Autodesk Fusion 360 part; units mm, degrees
note: some values were not read from the file. Set by a fixed rule: which sketch regions a step uses.
(part 3 of 8)
  line L1327 (107.274, 60.7841) -> (107.274, 61.6082)
  line L1328 (90.83, 67.0833) -> (104.831, 67.0833)
  line L1329 (38.442, 33.0844) -> (37.642, 33.0844)
  line L1330 (124.167, 80.0836) -> (123.367, 80.0836)
  line L1331 (100.355, 105.5592) -> (99.556, 105.5592)
  line L1332 (80.506, 108.6602) -> (81.305, 108.6602)
  line L1333 (138.167, 81.084) -> (124.167, 81.084)
  line L1334 (124.167, 76.9844) -> (123.367, 76.9844)
  line L1335 (38.442, 38.8844) -> (37.642, 38.8844)
  line L1336 (95.306, 108.6602) -> (96.105, 108.6602)
  line L1337 (81.305, 99.7592) -> (80.506, 99.7592)
  line L1338 (37.642, 38.8844) -> (37.642, 41.9836)
  line L1339 (115.155, 108.6602) -> (114.356, 108.6602)
  line L1340 (80.506, 105.5592) -> (81.305, 105.5592)
  line L1341 (100.355, 109.6602) -> (114.356, 109.6602)
  line L1342 (142.417, 105.5592) -> (143.217, 105.5592)
  line L1343 (123.367, 68.0838) -> (123.367, 71.1844)
  line L1344 (37.642, 41.9836) -> (37.642, 38.8844)
  line L1345 (95.306, 108.6602) -> (95.306, 109.6602)
  line L1346 (81.305, 96.6592) -> (81.305, 95.6582)
  line L1347 (38.442, 29.9838) -> (37.642, 29.9838)
  line L1348 (100.355, 108.6602) -> (100.355, 109.6602)
  line L1349 (96.105, 108.6602) -> (96.105, 105.5592)
  line L1350 (90.031, 71.1844) -> (90.83, 71.1844)
  arc A24 (90.274, 120.9832) -> (88.274, 118.9832) centre (90.274, 118.9832) ccw
  line L1351 (110.974, 53.3084) -> (110.974, 52.509)
  line L1352 (90.031, 68.0838) -> (90.031, 71.1844)
  line L1353 (95.306, 109.6602) -> (95.306, 108.6602)
  line L1354 (96.105, 105.5592) -> (95.306, 105.5592)
  line L1355 (80.506, 99.7592) -> (80.506, 96.6592)
  line L1356 (100.355, 109.6602) -> (100.355, 108.6602)
  circle A25 centre (99.974, 117.5832) radius 1.7
  arc A26 (86.274, 114.1832) -> (88.274, 116.1832) centre (86.274, 116.1832) ccw
  line L1357 (81.305, 96.6592) -> (80.506, 96.6592)
  line L1358 (81.305, 95.6582) -> (81.305, 96.6592)
  line L1359 (115.155, 108.6602) -> (115.155, 105.5592)
  line L1360 (138.968, 96.6592) -> (138.968, 99.7592)
  line L1361 (89.306, 67.3134) -> (87.581, 67.3134)
  line L1362 (90.83, 71.1844) -> (90.83, 71.7838)
  line L1363 (100.355, 108.6602) -> (99.556, 108.6602)
  line L1364 (102.673, 52.509) -> (102.673, 54.0334)
  line L1365 (114.356, 109.6602) -> (100.355, 109.6602)
  line L1366 (90.83, 67.0833) -> (90.83, 68.0838)
  line L1367 (104.474, 61.6082) -> (104.474, 60.7841)
  line L1368 (43.718, 22.9336) -> (42.917, 22.9336)
  line L1369 (97.974, 52.509) -> (98.973, 52.509)
  line L1370 (90.031, 71.1844) -> (90.031, 68.0838)
  line L1371 (43.718, 22.9336) -> (43.718, 19.8345)
  line L1372 (111.674, 118.9832) -> (111.674, 116.1832)
  line L1373 (90.83, 71.7838) -> (89.306, 71.7838)
  line L1374 (81.305, 108.6602) -> (81.305, 109.6602)
  line L1375 (42.917, 22.9336) -> (42.917, 23.934)
  line L1376 (98.204, 59.0591) -> (98.204, 60.7841)
  line L1377 (138.968, 108.6602) -> (138.968, 105.5592)
  line L1378 (81.305, 99.7592) -> (81.305, 105.5592)
  line L1379 (98.204, 59.0591) -> (97.224, 59.0591)
  line L1380 (28.117, 22.9336) -> (28.917, 22.9336)
  line L1381 (90.031, 68.0838) -> (90.83, 68.0838)
  line L1382 (143.217, 108.6602) -> (143.217, 109.6602)
  line L1383 (81.305, 108.6602) -> (80.506, 108.6602)
  line L1384 (80.506, 99.7592) -> (81.305, 99.7592)
  line L1385 (109.674, 120.9832) -> (90.274, 120.9832)
  line L1386 (81.305, 109.6602) -> (81.305, 108.6602)
  line L1387 (80.506, 108.6602) -> (80.506, 105.5592)
  line L1388 (87.581, 66.3337) -> (87.581, 67.3134)
  line L1389 (142.417, 96.6592) -> (143.217, 96.6592)
  line L1390 (114.356, 105.5592) -> (115.155, 105.5592)
  line L1391 (95.306, 105.5592) -> (96.105, 105.5592)
  line L1392 (138.167, 105.5592) -> (138.968, 105.5592)
  line L1393 (114.356, 108.6602) -> (114.356, 109.6602)
  line L1394 (104.474, 60.7841) -> (98.204, 60.7841)
  line L1395 (138.968, 108.6602) -> (138.167, 108.6602)
  line L1396 (95.306, 95.6582) -> (81.305, 95.6582)
  line L1397 (96.105, 108.6602) -> (95.306, 108.6602)
  line L1398 (28.917, 23.934) -> (28.917, 22.9336)
  arc A27 (181.673, -20.7426) -> (183.673, -18.7426) centre (181.673, -18.7426) ccw
  line L1399 (80.506, 96.6592) -> (81.305, 96.6592)
  arc A28 (224.567, -18.7426) -> (226.567, -20.7426) centre (226.567, -18.7426) ccw
  line L1400 (89.306, 67.3134) -> (89.306, 71.7838)
  circle A29 centre (171.973, -17.3426) radius 1.7
  line L1401 (90.83, 68.0838) -> (90.83, 67.0833)
  line L1402 (138.167, 95.6582) -> (138.167, 96.6592)
  line L1403 (102.673, 52.509) -> (102.073, 52.509)
  line L1404 (143.217, 68.0838) -> (143.217, 67.0833)
  line L1405 (138.167, 96.6592) -> (138.968, 96.6592)
  line L1406 (99.556, 105.5592) -> (99.556, 108.6602)
  line L1407 (84.28, 66.3337) -> (87.581, 66.3337)
  line L1408 (89.306, 71.7838) -> (89.306, 67.3134)
  line L1409 (42.917, 19.8345) -> (43.718, 19.8345)
  line L1410 (43.718, 19.8345) -> (42.917, 19.8345)
  line L1411 (143.217, 108.6602) -> (142.417, 108.6602)
  line L1412 (100.374, 120.9832) -> (99.574, 120.9832)
  line L1413 (98.973, 52.509) -> (98.973, 53.3084)
  line L1414 (88.274, 118.9832) -> (88.274, 116.1832)
  line L1415 (28.917, 22.9336) -> (28.117, 22.9336)
  arc A30 (245.967, -20.7426) -> (247.967, -18.7426) centre (245.967, -18.7426) ccw
  line L1416 (87.581, 66.3337) -> (84.28, 66.3337)
  line L1417 (96.105, 105.5592) -> (96.105, 108.6602)
  line L1418 (42.917, 23.934) -> (42.917, 22.9336)
  line L1419 (143.217, 109.6602) -> (143.217, 108.6602)
  line L1420 (142.417, 71.1844) -> (142.417, 68.0838)
  arc A31 (160.273, -15.9426) -> (158.273, -13.9426) centre (158.273, -15.9426) ccw
  line L1421 (81.305, 95.6582) -> (95.306, 95.6582)
  line L1422 (87.581, 67.3134) -> (87.581, 66.3337)
  line L1423 (81.731, 76.3836) -> (82.555, 76.3836)
  line L1424 (47.681, 61.0336) -> (47.681, 62.034)
  line L1425 (82.555, 67.3134) -> (84.28, 67.3134)
  line L1426 (24.668, 22.9336) -> (24.668, 19.8345)
  line L1427 (51.931, 49.0338) -> (52.73, 49.0338)
  line L1428 (-119.0079, 28.9833) -> (-133.0076, 28.9833)
  line L1429 (24.668, 19.8345) -> (23.867, 19.8345)
  line L1430 (48.48, 52.1344) -> (47.681, 52.1344)
  line L1431 (23.867, 22.9336) -> (23.867, 23.934)
  line L1432 (82.555, 79.6137) -> (82.555, 76.3836)
  line L1433 (8.724, 0.1836) -> (-30.902, 0.1836)
  arc A32 (-163.6637, -15.9426) -> (-165.6637, -13.9426) centre (-165.6637, -15.9426) ccw
  line L1434 (24.668, 22.9336) -> (23.867, 22.9336)
  arc A33 (-147.2637, -20.7426) -> (-145.2637, -18.7426) centre (-147.2637, -18.7426) ccw
  line L1435 (-18.994, 81.084) -> (-32.995, 81.084)
  line L1436 (23.867, 19.8345) -> (24.668, 19.8345)
  line L1437 (47.681, 52.1344) -> (47.681, 57.9344)
  line L1438 (77.055, 68.0838) -> (77.055, 71.1844)
  line L1439 (47.681, 61.0336) -> (48.48, 61.0336)
  line L1440 (-140.1512, -9.1167) -> (-126.1517, -9.1167)
  line L1441 (-145.2637, -18.7426) -> (-145.2637, -15.9426)
  line L1442 (76.256, 71.1844) -> (76.256, 76.9844)
  arc A34 (-106.601, -18.7426) -> (-104.601, -20.7426) centre (-104.601, -18.7426) ccw
  line L1443 (24.668, 19.8345) -> (24.668, 22.9336)
  line L1444 (-133.0076, 28.9833) -> (-119.0079, 28.9833)
  line L1445 (81.731, 73.5836) -> (82.555, 73.5836)
  line L1446 (51.931, 57.9344) -> (51.931, 61.0336)
  line L1447 (77.055, 80.0836) -> (76.256, 80.0836)
  line L1448 (-23.47, 62.034) -> (-9.469, 62.034)
  line L1449 (23.867, 23.934) -> (23.867, 22.9336)
  line L1450 (81.731, 76.3836) -> (81.731, 73.5836)
  arc A35 (-106.601, -15.9426) -> (-108.601, -13.9426) centre (-108.601, -15.9426) ccw
  line L1451 (-142.5325, 23.934) -> (-128.5329, 23.934)
  circle A36 centre (-156.9637, -17.3426) radius 1.7
  line L1452 (-18.994, 67.0833) -> (-32.995, 67.0833)
  line L1453 (-128.5329, 9.9333) -> (-142.5325, 9.9333)
  circle A37 centre (-156.9637, -17.3426) radius 1.7
  line L1454 (19.392, 42.984) -> (33.392, 42.984)
  line L1455 (-165.6637, -13.9426) -> (-171.0689, -13.9426)
  arc A38 (-163.6637, -18.7426) -> (-161.6637, -20.7426) centre (-161.6637, -18.7426) ccw
  line L1456 (-123.769, 62.034) -> (-137.77, 62.034)
  line L1457 (28.631, 57.9344) -> (29.43, 57.9344)
  line L1458 (23.867, 22.9336) -> (24.668, 22.9336)
  line L1459 (-4.708, 28.9833) -> (-18.708, 28.9833)
  line L1460 (-126.1517, -9.1167) -> (-140.1512, -9.1167)
  line L1461 (-32.995, 67.0833) -> (-18.994, 67.0833)
  line L1462 (261.656, -7.9426) -> (261.656, 108.1832)
  circle A39 centre (-94.901, -17.3426) radius 1.7
  line L1463 (-126.1517, 4.8841) -> (-140.1512, 4.8841)
  line L1464 (28.631, 49.0338) -> (28.631, 48.0333)
  line L1465 (-133.0076, 42.984) -> (-119.0079, 42.984)
  line L1466 (-119.0079, 42.984) -> (-133.0076, 42.984)
  line L1467 (19.392, 28.9833) -> (33.392, 28.9833)
  line L1468 (33.392, 28.9833) -> (19.392, 28.9833)
  line L1469 (33.392, 42.984) -> (19.392, 42.984)
  line L1470 (-18.708, 42.984) -> (-4.708, 42.984)
  line L1471 (-114.244, 67.0833) -> (-128.2451, 67.0833)
  arc A40 (-143.2637, -13.9426) -> (-145.2637, -15.9426) centre (-143.2637, -15.9426) ccw
  line L1472 (29.43, 49.0338) -> (28.631, 49.0338)
  line L1473 (5.398, -13.9426) -> (-81.201, -13.9426)
  line L1474 (33.68, 52.1344) -> (33.68, 57.9344)
  line L1475 (-108.601, -13.9426) -> (-143.2637, -13.9426)
  line L1476 (-150.5637, -13.9426) -> (-101.301, -13.9426)
  circle A41 centre (-94.901, -17.3426) radius 1.7
  line L1477 (-106.601, -18.7426) -> (-106.601, -15.9426)
  line L1478 (195.605, -9.1167) -> (209.607, -9.1167)
  line L1479 (219.132, 41.9836) -> (219.132, 42.984)
  line L1480 (157.217, 22.9336) -> (157.217, 23.934)
  line L1481 (0.342, 29.9838) -> (0.342, 28.9833)
  line L1482 (32.881, 52.1344) -> (33.68, 52.1344)
  line L1483 (28.631, 61.0336) -> (28.631, 62.034)
  line L1484 (158.018, 22.9336) -> (157.217, 22.9336)
  line L1485 (32.881, 57.9344) -> (32.881, 61.0336)
  line L1486 (28.631, 52.1344) -> (29.43, 52.1344)
  line L1487 (-95.301, -20.7426) -> (-94.501, -20.7426)
  line L1488 (-163.6637, -18.7426) -> (-163.6637, -15.9426)
  line L1489 (32.881, 52.1344) -> (32.881, 49.0338)
  line L1490 (157.217, 14.0343) -> (157.217, 19.8345)
  line L1491 (29.43, 49.0338) -> (29.43, 52.1344)
  line L1492 (32.881, 57.9344) -> (33.68, 57.9344)
  line L1493 (185.673, 114.1832) -> (222.567, 114.1832)
  line L1494 (157.217, 22.9336) -> (158.018, 22.9336)
  line L1495 (157.217, 14.0343) -> (158.018, 14.0343)
  line L1496 (29.43, 52.1344) -> (28.631, 52.1344)
  line L1497 (-114.244, 81.084) -> (-128.2451, 81.084)
  line L1498 (158.018, 19.8345) -> (158.018, 22.9336)
  line L1499 (33.68, 48.0333) -> (33.68, 49.0338)
  line L1500 (0.342, 38.8844) -> (0.342, 33.0844)
  line L1501 (158.018, 14.0343) -> (158.018, 10.9337)
  line L1502 (32.881, 49.0338) -> (33.68, 49.0338)
  line L1503 (157.217, 10.9337) -> (158.018, 10.9337)
  line L1504 (-9.469, 95.6582) -> (-23.47, 95.6582)
  line L1505 (219.132, 33.0844) -> (219.132, 38.8844)
  line L1506 (29.43, 57.9344) -> (29.43, 61.0336)
  line L1507 (-99.6701, 62.034) -> (-99.6701, 61.0336)
  line L1508 (238.182, -9.1167) -> (224.18, -9.1167)
  line L1509 (32.881, 49.0338) -> (32.881, 52.1344)
  line L1510 (-100.4691, 61.0336) -> (-100.4691, 57.9344)
  line L1511 (158.018, 19.8345) -> (157.217, 19.8345)
  line L1512 (-9.469, 62.034) -> (-23.47, 62.034)
  line L1513 (186.08, 33.0844) -> (185.279, 33.0844)
  line L1514 (-0.458, 29.9838) -> (0.342, 29.9838)
  line L1515 (158.018, 10.9337) -> (157.217, 10.9337)
  line L1516 (-103.92, 52.1344) -> (-103.92, 49.0338)
  line L1517 (158.018, 10.9337) -> (158.018, 14.0343)
  line L1518 (-103.92, 49.0338) -> (-103.92, 52.1344)
  line L1519 (0.342, 42.984) -> (0.342, 41.9836)
  line L1520 (219.132, 38.8844) -> (219.132, 33.0844)
  line L1521 (158.018, 22.9336) -> (158.018, 19.8345)
  line L1522 (157.217, 23.934) -> (157.217, 22.9336)
  line L1523 (28.631, 49.0338) -> (29.43, 49.0338)
  line L1524 (161.467, 61.0336) -> (161.467, 57.9344)
  line L1525 (186.08, 38.8844) -> (185.279, 38.8844)
  line L1526 (-100.4691, 57.9344) -> (-100.4691, 61.0336)
  line L1527 (-103.92, 57.9344) -> (-103.92, 61.0336)
  line L1528 (194.804, 3.8837) -> (194.804, 0.7845)
  line L1529 (32.881, 61.0336) -> (32.881, 57.9344)
  line L1530 (29.43, 61.0336) -> (29.43, 57.9344)
  line L1531 (-0.458, 38.8844) -> (-0.458, 41.9836)
  line L1532 (-28.233, 9.9333) -> (-14.233, 9.9333)
  line L1533 (0.342, 29.9838) -> (-0.458, 29.9838)
  line L1534 (0.342, 33.0844) -> (-0.458, 33.0844)
  line L1535 (192.356, 4.3343) -> (192.356, 3.4138)
  line L1536 (161.467, 49.0338) -> (161.467, 52.1344)
  line L1537 (-104.719, 48.0333) -> (-104.719, 49.0338)
  line L1538 (-100.4691, 52.1344) -> (-100.4691, 49.0338)
  line L1539 (33.68, 49.0338) -> (33.68, 48.0333)
  line L1540 (157.217, 49.0338) -> (157.217, 48.0333)
  line L1541 (158.018, 49.0338) -> (158.018, 52.1344)
  line L1542 (157.217, 19.8345) -> (158.018, 19.8345)
  line L1543 (-103.92, 61.0336) -> (-103.92, 57.9344)
  line L1544 (157.217, 10.9337) -> (157.217, 9.9333)
  line L1545 (185.279, 38.8844) -> (185.279, 41.9836)
  line L1546 (157.217, 9.9333) -> (157.217, 10.9337)
  line L1547 (-0.458, 41.9836) -> (0.342, 41.9836)
  line L1548 (33.68, 57.9344) -> (33.68, 52.1344)
  line L1549 (-0.458, 33.0844) -> (-0.458, 29.9838)
  line L1550 (33.68, 61.0336) -> (32.881, 61.0336)
  line L1551 (157.217, 48.0333) -> (157.217, 49.0338)
  line L1552 (-0.458, 41.9836) -> (-0.458, 38.8844)
  line L1553 (28.631, 61.0336) -> (29.43, 61.0336)
  line L1554 (-100.4691, 52.1344) -> (-99.6701, 52.1344)
  line L1555 (192.356, 3.4138) -> (192.356, 4.3343)
  line L1556 (157.217, 19.8345) -> (157.217, 14.0343)
  line L1557 (0.342, 33.0844) -> (0.342, 38.8844)
  line L1558 (194.081, 3.4138) -> (194.081, 0.1836)
  line L1559 (158.018, 14.0343) -> (157.217, 14.0343)
  line L1560 (189.054, 4.3343) -> (189.054, 3.4138)
  line L1561 (32.881, 61.0336) -> (33.68, 61.0336)
  line L1562 (157.217, 61.0336) -> (157.217, 62.034)
  line L1563 (158.018, 61.0336) -> (157.217, 61.0336)
  line L1564 (189.054, 4.3343) -> (192.356, 4.3343)
  line L1565 (157.217, 57.9344) -> (158.018, 57.9344)
  line L1566 (-0.458, 29.9838) -> (-0.458, 33.0844)
  line L1567 (0.342, 41.9836) -> (0.342, 42.984)
  line L1568 (-100.4691, 61.0336) -> (-99.6701, 61.0336)
  line L1569 (-99.6701, 52.1344) -> (-100.4691, 52.1344)
  line L1570 (186.08, 41.9836) -> (185.279, 41.9836)
  line L1571 (-0.458, 33.0844) -> (0.342, 33.0844)
  line L1572 (162.267, 61.0336) -> (161.467, 61.0336)
  line L1573 (162.267, -9.1167) -> (176.267, -9.1167)
  line L1574 (-99.6701, 48.0333) -> (-99.6701, 49.0338)
  line L1575 (29.43, 61.0336) -> (28.631, 61.0336)
  line L1576 (162.267, 4.8841) -> (176.267, 4.8841)
  line L1577 (186.08, 42.984) -> (186.08, 41.9836)
  line L1578 (33.68, 52.1344) -> (32.881, 52.1344)
  line L1579 (187.329, 3.4138) -> (187.329, 0.1836)
  line L1580 (186.08, 28.9833) -> (186.08, 29.9838)
  line L1581 (29.43, 57.9344) -> (28.631, 57.9344)
  line L1582 (162.267, 61.0336) -> (162.267, 62.034)
  line L1583 (-9.469, 109.6602) -> (-23.47, 109.6602)
  line L1584 (186.08, 10.9337) -> (186.08, 9.9333)
  line L1585 (157.217, 52.1344) -> (158.018, 52.1344)
  line L1586 (-0.458, 38.8844) -> (0.342, 38.8844)
  line L1587 (186.08, 14.0343) -> (185.279, 14.0343)
  line L1588 (-104.719, 57.9344) -> (-103.92, 57.9344)
  line L1589 (194.081, 3.4138) -> (192.356, 3.4138)
  line L1590 (-14.233, 23.934) -> (-28.233, 23.934)
  line L1591 (185.279, 33.0844) -> (186.08, 33.0844)
  line L1592 (0.342, 38.8844) -> (-0.458, 38.8844)
  line L1593 (223.379, 41.9836) -> (223.379, 38.8844)
  line L1594 (-99.6701, 49.0338) -> (-99.6701, 48.0333)
  line L1595 (186.08, 29.9838) -> (185.279, 29.9838)
  line L1596 (-23.47, 109.6602) -> (-9.469, 109.6602)
  line L1597 (-99.6701, 61.0336) -> (-99.6701, 62.034)
  line L1598 (143.217, 96.6592) -> (143.217, 95.6582)
  line L1599 (57.206, 108.6602) -> (58.005, 108.6602)
  line L1600 (104.831, 81.084) -> (90.83, 81.084)
  line L1601 (77.055, 96.6592) -> (76.256, 96.6592)
  line L1602 (90.83, 76.9844) -> (90.031, 76.9844)
  line L1603 (76.256, 99.7592) -> (76.256, 105.5592)
  line L1604 (142.417, 68.0838) -> (143.217, 68.0838)
  line L1605 (143.217, 99.7592) -> (143.217, 105.5592)
  line L1606 (138.167, 68.0838) -> (138.167, 67.0833)
  line L1607 (76.256, 95.6582) -> (76.256, 96.6592)
  line L1608 (76.256, 105.5592) -> (76.256, 99.7592)
  line L1609 (138.167, 76.9844) -> (138.968, 76.9844)
  line L1610 (89.306, 76.3836) -> (90.83, 76.3836)
  line L1611 (90.031, 76.9844) -> (90.031, 80.0836)
  line L1612 (61.456, 96.6592) -> (61.456, 99.7592)
  line L1613 (138.968, 80.0836) -> (138.167, 80.0836)
  line L1614 (58.005, 108.6602) -> (58.005, 105.5592)
  line L1615 (90.83, 76.3836) -> (90.83, 76.9844)
  line L1616 (87.581, 80.5344) -> (87.581, 79.6137)
  line L1617 (77.055, 108.6602) -> (76.256, 108.6602)
  line L1618 (57.206, 96.6592) -> (58.005, 96.6592)
  line L1619 (90.031, 76.9844) -> (90.83, 76.9844)
  line L1620 (77.055, 99.7592) -> (77.055, 96.6592)
  line L1621 (90.83, 81.084) -> (104.831, 81.084)
  line L1622 (87.581, 80.5344) -> (84.28, 80.5344)
  line L1623 (62.255, 67.0833) -> (76.256, 67.0833)
  line L1624 (138.968, 76.9844) -> (138.968, 80.0836)
  line L1625 (90.83, 76.9844) -> (90.83, 76.3836)
  line L1626 (18.592, 33.0844) -> (18.592, 29.9838)
  line L1627 (15.143, 41.9836) -> (14.342, 41.9836)
  line L1628 (76.256, 108.6602) -> (76.256, 109.6602)
  line L1629 (66.731, 48.0333) -> (52.73, 48.0333)
  line L1630 (14.342, 38.8844) -> (14.342, 33.0844)
  line L1631 (77.055, 105.5592) -> (77.055, 108.6602)
  line L1632 (142.417, 80.0836) -> (143.217, 80.0836)
  line L1633 (-76.144, 109.6602) -> (-90.1451, 109.6602)
  line L1634 (90.83, 81.084) -> (90.83, 80.0836)
  line L1635 (90.83, 76.3836) -> (89.306, 76.3836)
  line L1636 (143.217, 76.9844) -> (142.417, 76.9844)
  line L1637 (138.968, 71.1844) -> (138.167, 71.1844)
  line L1638 (14.342, 33.0844) -> (15.143, 33.0844)
  line L1639 (52.73, 48.0333) -> (66.731, 48.0333)
  line L1640 (90.83, 80.0836) -> (90.031, 80.0836)
  line L1641 (142.417, 71.1844) -> (143.217, 71.1844)
  line L1642 (57.206, 81.084) -> (57.206, 80.0836)
  line L1643 (89.306, 79.6137) -> (87.581, 79.6137)
  line L1644 (61.456, 105.5592) -> (62.255, 105.5592)
  line L1645 (77.055, 99.7592) -> (76.256, 99.7592)
  line L1646 (19.392, 33.0844) -> (18.592, 33.0844)
  line L1647 (142.417, 68.0838) -> (142.417, 71.1844)
  line L1648 (62.255, 95.6582) -> (62.255, 96.6592)
  line L1649 (104.831, 67.0833) -> (90.83, 67.0833)
  line L1650 (52.73, 62.034) -> (66.731, 62.034)
  line L1651 (138.968, 68.0838) -> (138.968, 71.1844)
  line L1652 (-85.201, 120.9832) -> (-104.601, 120.9832)
  line L1653 (14.342, 38.8844) -> (15.143, 38.8844)
  line L1654 (66.731, 52.1344) -> (67.53, 52.1344)
  line L1655 (90.83, 80.0836) -> (90.83, 81.084)
  line L1656 (57.206, 99.7592) -> (58.005, 99.7592)
  line L1657 (142.417, 80.0836) -> (142.417, 76.9844)
  line L1658 (19.392, 29.9838) -> (18.592, 29.9838)
  line L1659 (82.555, 79.6137) -> (84.28, 79.6137)
  line L1660 (18.592, 38.8844) -> (18.592, 41.9836)
  line L1661 (67.53, 57.9344) -> (67.53, 61.0336)
  line L1662 (76.256, 76.9844) -> (77.055, 76.9844)
  line L1663 (14.342, 29.9838) -> (15.143, 29.9838)
  line L1664 (66.731, 62.034) -> (52.73, 62.034)
  line L1665 (138.167, 81.084) -> (138.167, 80.0836)
  line L1666 (138.167, 80.0836) -> (138.968, 80.0836)
  line L1667 (143.217, 81.084) -> (143.217, 80.0836)
  line L1668 (58.005, 96.6592) -> (58.005, 99.7592)
  line L1669 (15.143, 29.9838) -> (14.342, 29.9838)
  line L1670 (58.005, 96.6592) -> (57.206, 96.6592)
  line L1671 (67.53, 49.0338) -> (66.731, 49.0338)
  line L1672 (18.592, 29.9838) -> (19.392, 29.9838)
  line L1673 (57.206, 71.1844) -> (57.206, 76.9844)
  line L1674 (104.831, 76.3836) -> (104.831, 76.9844)
  line L1675 (57.206, 109.6602) -> (57.206, 108.6602)
  line L1676 (15.143, 29.9838) -> (15.143, 33.0844)
  line L1677 (52.73, 57.9344) -> (52.73, 52.1344)
  line L1678 (76.256, 80.0836) -> (77.055, 80.0836)
  line L1679 (104.831, 80.0836) -> (104.831, 81.084)
  line L1680 (67.53, 52.1344) -> (67.53, 49.0338)
  line L1681 (138.167, 68.0838) -> (138.968, 68.0838)
  line L1682 (104.831, 81.084) -> (104.831, 80.0836)
  line L1683 (89.306, 76.3836) -> (89.306, 79.6137)
  line L1684 (66.731, 61.0336) -> (66.731, 62.034)
  line L1685 (143.217, 71.1844) -> (142.417, 71.1844)
  line L1686 (61.456, 99.7592) -> (62.255, 99.7592)
  line L1687 (143.217, 68.0838) -> (142.417, 68.0838)
  line L1688 (57.206, 99.7592) -> (57.206, 105.5592)
  line L1689 (81.731, 73.5836) -> (81.731, 76.3836)
  line L1690 (58.005, 108.6602) -> (57.206, 108.6602)
  line L1691 (66.731, 62.034) -> (66.731, 61.0336)
  line L1692 (15.143, 38.8844) -> (14.342, 38.8844)
  line L1693 (57.206, 80.0836) -> (57.206, 81.084)
  line L1694 (14.342, 41.9836) -> (14.342, 42.984)
  line L1695 (138.167, 71.1844) -> (138.968, 71.1844)
  line L1696 (62.255, 76.9844) -> (62.255, 71.1844)
  line L1697 (58.005, 76.9844) -> (57.206, 76.9844)
  line L1698 (61.456, 96.6592) -> (62.255, 96.6592)
  line L1699 (62.255, 99.7592) -> (61.456, 99.7592)
  line L1700 (67.53, 49.0338) -> (67.53, 52.1344)
  line L1701 (62.255, 105.5592) -> (61.456, 105.5592)
  line L1702 (52.73, 48.0333) -> (52.73, 49.0338)
  line L1703 (47.681, 48.0333) -> (47.681, 49.0338)
  line L1704 (57.206, 108.6602) -> (57.206, 109.6602)
  line L1705 (67.53, 61.0336) -> (67.53, 57.9344)
  line L1706 (58.005, 99.7592) -> (57.206, 99.7592)
  line L1707 (84.28, 79.6137) -> (84.28, 80.5344)
  line L1708 (66.731, 61.0336) -> (67.53, 61.0336)
  line L1709 (138.968, 71.1844) -> (138.968, 68.0838)
  line L1710 (62.255, 96.6592) -> (61.456, 96.6592)
  line L1711 (57.206, 76.9844) -> (58.005, 76.9844)
  line L1712 (138.968, 80.0836) -> (138.968, 76.9844)
  line L1713 (67.53, 52.1344) -> (66.731, 52.1344)
  line L1714 (19.392, 41.9836) -> (19.392, 42.984)
  line L1715 (61.456, 76.9844) -> (61.456, 80.0836)
  line L1716 (15.143, 33.0844) -> (15.143, 29.9838)
  line L1717 (61.456, 68.0838) -> (62.255, 68.0838)
  line L1718 (138.167, 76.9844) -> (138.167, 71.1844)
  line L1719 (18.592, 41.9836) -> (18.592, 38.8844)
  line L1720 (57.206, 96.6592) -> (57.206, 95.6582)
  line L1721 (14.342, 33.0844) -> (14.342, 38.8844)
  line L1722 (61.456, 71.1844) -> (61.456, 68.0838)
  line L1723 (19.392, 38.8844) -> (18.592, 38.8844)
  line L1724 (67.53, 57.9344) -> (66.731, 57.9344)
  line L1725 (61.456, 108.6602) -> (61.456, 105.5592)
  line L1726 (57.206, 68.0838) -> (58.005, 68.0838)
  line L1727 (62.255, 71.1844) -> (61.456, 71.1844)
  line L1728 (62.255, 80.0836) -> (61.456, 80.0836)
  line L1729 (18.592, 33.0844) -> (19.392, 33.0844)
  line L1730 (61.456, 99.7592) -> (61.456, 96.6592)
  line L1731 (62.255, 108.6602) -> (61.456, 108.6602)
  line L1732 (58.005, 80.0836) -> (57.206, 80.0836)
  line L1733 (66.731, 52.1344) -> (66.731, 57.9344)
  line L1734 (61.456, 108.6602) -> (62.255, 108.6602)
  line L1735 (14.342, 41.9836) -> (15.143, 41.9836)
  line L1736 (77.055, 76.9844) -> (77.055, 80.0836)
  line L1737 (57.206, 105.5592) -> (58.005, 105.5592)
  line L1738 (66.731, 57.9344) -> (66.731, 52.1344)
  line L1739 (67.53, 61.0336) -> (66.731, 61.0336)
  line L1740 (62.255, 68.0838) -> (61.456, 68.0838)
  line L1741 (52.73, 52.1344) -> (52.73, 57.9344)
  line L1742 (61.456, 105.5592) -> (61.456, 108.6602)
  line L1743 (62.255, 76.9844) -> (61.456, 76.9844)
  line L1744 (57.206, 95.6582) -> (57.206, 96.6592)
  line L1745 (18.592, 29.9838) -> (18.592, 33.0844)
  line L1746 (66.731, 57.9344) -> (67.53, 57.9344)
  line L1747 (58.005, 105.5592) -> (58.005, 108.6602)
  line L1748 (57.206, 105.5592) -> (57.206, 99.7592)
  line L1749 (47.681, 57.9344) -> (48.48, 57.9344)
  line L1750 (48.48, 49.0338) -> (48.48, 52.1344)
  line L1751 (77.055, 71.1844) -> (76.256, 71.1844)
  line L1752 (15.143, 41.9836) -> (15.143, 38.8844)
  line L1753 (62.255, 80.0836) -> (62.255, 81.084)
  line L1754 (19.392, 33.0844) -> (19.392, 38.8844)
  line L1755 (61.456, 76.9844) -> (62.255, 76.9844)
  line L1756 (82.555, 73.5836) -> (82.555, 67.3134)
  line L1757 (19.392, 29.9838) -> (19.392, 28.9833)
  line L1758 (52.73, 49.0338) -> (51.931, 49.0338)
  line L1759 (62.255, 68.0838) -> (62.255, 67.0833)
  line L1760 (58.005, 105.5592) -> (57.206, 105.5592)
  line L1761 (62.255, 71.1844) -> (62.255, 76.9844)
  line L1762 (15.143, 33.0844) -> (14.342, 33.0844)
  line L1763 (61.456, 71.1844) -> (62.255, 71.1844)
  line L1764 (76.256, 81.084) -> (76.256, 80.0836)
  line L1765 (52.73, 61.0336) -> (52.73, 62.034)
  line L1766 (51.931, 52.1344) -> (51.931, 49.0338)
  line L1767 (61.456, 80.0836) -> (61.456, 76.9844)
  line L1768 (15.143, 38.8844) -> (15.143, 41.9836)
  line L1769 (66.731, 49.0338) -> (66.731, 48.0333)
  line L1770 (57.206, 80.0836) -> (58.005, 80.0836)
  line L1771 (52.73, 62.034) -> (52.73, 61.0336)
  line L1772 (52.73, 61.0336) -> (51.931, 61.0336)
  line L1773 (48.48, 61.0336) -> (47.681, 61.0336)
  line L1774 (-171.0689, -13.9426) -> (-171.0689, 114.1832)
  line L1775 (52.73, 52.1344) -> (51.931, 52.1344)
  line L1776 (57.206, 76.9844) -> (57.206, 71.1844)
  line L1777 (82.555, 76.3836) -> (81.731, 76.3836)
  line L1778 (76.256, 67.0833) -> (76.256, 68.0838)
  line L1779 (58.005, 99.7592) -> (58.005, 96.6592)
  line L1780 (77.055, 68.0838) -> (76.256, 68.0838)
  line L1781 (58.005, 68.0838) -> (57.206, 68.0838)
  line L1782 (62.255, 109.6602) -> (62.255, 108.6602)
  line L1783 (47.681, 62.034) -> (47.681, 61.0336)
  line L1784 (77.055, 71.1844) -> (77.055, 68.0838)
  line L1785 (84.28, 66.3337) -> (84.28, 67.3134)
  line L1786 (76.256, 80.0836) -> (76.256, 81.084)
  line L1787 (19.392, 41.9836) -> (18.592, 41.9836)
  line L1788 (84.28, 67.3134) -> (84.28, 66.3337)
  line L1789 (82.555, 67.3134) -> (82.555, 73.5836)
  line L1790 (14.342, 28.9833) -> (14.342, 29.9838)
  line L1791 (82.555, 73.5836) -> (81.731, 73.5836)
  line L1792 (-30.902, -4.4162) -> (8.724, -4.4162)
  line L1793 (58.005, 71.1844) -> (58.005, 68.0838)
  line L1794 (66.731, 48.0333) -> (66.731, 49.0338)
  line L1795 (57.206, 67.0833) -> (57.206, 68.0838)
  line L1796 (62.255, 81.084) -> (62.255, 80.0836)
  line L1797 (51.931, 49.0338) -> (51.931, 52.1344)
  line L1798 (47.681, 57.9344) -> (47.681, 52.1344)
  line L1799 (62.255, 67.0833) -> (62.255, 68.0838)
  line L1800 (52.73, 49.0338) -> (52.73, 48.0333)
  line L1801 (47.681, 49.0338) -> (48.48, 49.0338)
  line L1802 (76.256, 76.9844) -> (76.256, 71.1844)
  line L1803 (48.48, 52.1344) -> (48.48, 49.0338)
  line L1804 (61.456, 68.0838) -> (61.456, 71.1844)
  line L1805 (47.681, 49.0338) -> (47.681, 48.0333)
  line L1806 (66.731, 49.0338) -> (67.53, 49.0338)
  line L1807 (19.392, 42.984) -> (19.392, 41.9836)
  line L1808 (18.592, 38.8844) -> (19.392, 38.8844)
  line L1809 (58.005, 71.1844) -> (57.206, 71.1844)
  line L1810 (58.005, 68.0838) -> (58.005, 71.1844)
  line L1811 (84.28, 67.3134) -> (82.555, 67.3134)
  line L1812 (57.206, 68.0838) -> (57.206, 67.0833)
  line L1813 (19.392, 38.8844) -> (19.392, 33.0844)
  line L1814 (48.48, 57.9344) -> (48.48, 61.0336)
  line L1815 (48.48, 61.0336) -> (48.48, 57.9344)
  line L1816 (84.28, 80.5344) -> (84.28, 79.6137)
  line L1817 (14.342, 29.9838) -> (14.342, 28.9833)
  line L1818 (61.456, 80.0836) -> (62.255, 80.0836)
  line L1819 (8.724, -4.4162) -> (-30.902, -4.4162)
  line L1820 (14.342, 42.984) -> (14.342, 41.9836)
  line L1821 (76.256, 68.0838) -> (77.055, 68.0838)
  line L1822 (51.931, 57.9344) -> (52.73, 57.9344)
  line L1823 (52.73, 57.9344) -> (51.931, 57.9344)
  line L1824 (51.931, 61.0336) -> (52.73, 61.0336)
  line L1825 (-161.6637, -20.7426) -> (-147.2637, -20.7426)
  line L1826 (18.592, 41.9836) -> (19.392, 41.9836)
  line L1827 (58.005, 76.9844) -> (58.005, 80.0836)
  line L1828 (82.555, 76.3836) -> (82.555, 79.6137)
  line L1829 (51.931, 52.1344) -> (52.73, 52.1344)
  line L1830 (-171.0689, 108.1832) -> (-171.0689, -7.9426)
  line L1831 (57.206, 71.1844) -> (58.005, 71.1844)
  line L1832 (77.055, 76.9844) -> (76.256, 76.9844)
  line L1833 (-32.995, 81.084) -> (-18.994, 81.084)
  line L1834 (-23.47, 95.6582) -> (-9.469, 95.6582)
  line L1835 (47.681, 52.1344) -> (48.48, 52.1344)
  line L1836 (48.48, 57.9344) -> (47.681, 57.9344)
  line L1837 (51.931, 61.0336) -> (51.931, 57.9344)
  line L1838 (-9.469, 48.0333) -> (-23.47, 48.0333)
  line L1839 (76.256, 71.1844) -> (77.055, 71.1844)
  line L1840 (58.005, 80.0836) -> (58.005, 76.9844)
  line L1841 (-18.708, 28.9833) -> (-4.708, 28.9833)
  line L1842 (19.392, 28.9833) -> (19.392, 29.9838)
  line L1843 (77.055, 80.0836) -> (77.055, 76.9844)
  line L1844 (84.28, 79.6137) -> (82.555, 79.6137)
  line L1845 (-14.233, 9.9333) -> (-28.233, 9.9333)
  line L1846 (76.256, 68.0838) -> (76.256, 67.0833)
  line L1847 (48.48, 49.0338) -> (47.681, 49.0338)
  line L1848 (157.217, 57.9344) -> (157.217, 52.1344)
  line L1849 (219.929, 38.8844) -> (219.132, 38.8844)
  line L1850 (219.929, 29.9838) -> (219.132, 29.9838)
  line L1851 (209.607, 4.8841) -> (195.605, 4.8841)
  line L1852 (0.342, 41.9836) -> (-0.458, 41.9836)
  line L1853 (-99.6701, 61.0336) -> (-100.4691, 61.0336)
  line L1854 (219.929, 33.0844) -> (219.929, 29.9838)
  line L1855 (161.467, -5.0157) -> (162.267, -5.0157)
  line L1856 (161.467, -8.1163) -> (161.467, -5.0157)
  line L1857 (29.43, 52.1344) -> (29.43, 49.0338)
  line L1858 (176.267, 4.8841) -> (162.267, 4.8841)
  line L1859 (185.279, 10.9337) -> (185.279, 14.0343)
  line L1860 (-99.6701, 57.9344) -> (-100.4691, 57.9344)
  line L1861 (33.68, 49.0338) -> (32.881, 49.0338)
  line L1862 (158.018, 57.9344) -> (157.217, 57.9344)
  line L1863 (28.631, 48.0333) -> (28.631, 49.0338)
  line L1864 (-104.719, 61.0336) -> (-104.719, 62.034)
  line L1865 (158.018, 0.7845) -> (157.217, 0.7845)
  line L1866 (187.329, 3.4138) -> (189.054, 3.4138)
  line L1867 (158.018, 49.0338) -> (157.217, 49.0338)
  line L1868 (186.08, 29.9838) -> (186.08, 28.9833)
  line L1869 (0.342, 28.9833) -> (0.342, 29.9838)
  line L1870 (-100.4691, 57.9344) -> (-99.6701, 57.9344)
  line L1871 (33.68, 57.9344) -> (32.881, 57.9344)
  line L1872 (-104.719, 52.1344) -> (-103.92, 52.1344)
  line L1873 (219.132, 41.9836) -> (219.929, 41.9836)
  line L1874 (219.132, 42.984) -> (219.132, 41.9836)
  line L1875 (185.279, 38.8844) -> (186.08, 38.8844)
  line L1876 (33.68, 62.034) -> (33.68, 61.0336)
  line L1877 (157.217, 52.1344) -> (157.217, 57.9344)
  line L1878 (194.081, 0.1836) -> (194.081, 3.4138)
  line L1879 (200.082, 41.9836) -> (200.082, 42.984)
  line L1880 (-103.92, 52.1344) -> (-104.719, 52.1344)
  line L1881 (28.631, 52.1344) -> (28.631, 57.9344)
  line L1882 (158.018, 52.1344) -> (157.217, 52.1344)
  line L1883 (185.279, 29.9838) -> (185.279, 33.0844)
  line L1884 (187.329, 0.1836) -> (187.329, 3.4138)
  line L1885 (162.267, 52.1344) -> (161.467, 52.1344)
  line L1886 (161.467, 0.7845) -> (162.267, 0.7845)
  line L1887 (185.279, 41.9836) -> (186.08, 41.9836)
  line L1888 (219.929, 33.0844) -> (219.132, 33.0844)
  line L1889 (-104.719, 49.0338) -> (-103.92, 49.0338)
  line L1890 (28.631, 57.9344) -> (28.631, 52.1344)
  line L1891 (219.929, 41.9836) -> (219.132, 41.9836)
  line L1892 (185.279, 14.0343) -> (186.08, 14.0343)
  line L1893 (161.467, 52.1344) -> (161.467, 49.0338)
  line L1894 (-104.719, 52.1344) -> (-104.719, 57.9344)
  line L1895 (189.054, 3.4138) -> (187.329, 3.4138)
  line L1896 (158.018, -5.0157) -> (157.217, -5.0157)
  line L1897 (4.817, 22.9336) -> (4.817, 23.934)
  line L1898 (161.467, 57.9344) -> (162.267, 57.9344)
  line L1899 (224.18, 41.9836) -> (223.379, 41.9836)
  line L1900 (200.082, 28.9833) -> (200.082, 29.9838)
  line L1901 (-103.92, 61.0336) -> (-104.719, 61.0336)
  line L1902 (28.631, 62.034) -> (28.631, 61.0336)
  line L1903 (162.267, -8.1163) -> (161.467, -8.1163)
  line L1904 (33.68, 61.0336) -> (33.68, 62.034)
  line L1905 (224.18, 41.9836) -> (224.18, 42.984)
  line L1906 (161.467, 52.1344) -> (162.267, 52.1344)
  line L1907 (200.082, 33.0844) -> (200.082, 38.8844)
  line L1908 (9.067, 19.8345) -> (9.067, 22.9336)
  line L1909 (-104.719, 62.034) -> (-104.719, 61.0336)
  line L1910 (194.804, 3.8837) -> (195.605, 3.8837)
  line L1911 (186.08, 38.8844) -> (186.08, 33.0844)
  line L1912 (189.054, 3.4138) -> (189.054, 4.3343)
  line L1913 (162.267, 0.7845) -> (161.467, 0.7845)
  line L1914 (185.279, 29.9838) -> (186.08, 29.9838)
  line L1915 (219.929, 41.9836) -> (219.929, 38.8844)
  line L1916 (194.804, 0.7845) -> (194.804, 3.8837)
  line L1917 (157.217, 61.0336) -> (158.018, 61.0336)
  line L1918 (9.067, 22.9336) -> (9.067, 19.8345)
  line L1919 (161.467, -5.0157) -> (161.467, -8.1163)
  line L1920 (-99.6701, 57.9344) -> (-99.6701, 52.1344)
  line L1921 (200.082, 42.984) -> (200.082, 41.9836)
  line L1922 (9.867, 19.8345) -> (9.067, 19.8345)
  line L1923 (-100.4691, 49.0338) -> (-100.4691, 52.1344)
  line L1924 (161.467, 3.8837) -> (161.467, 0.7845)
  line L1925 (9.067, 19.8345) -> (9.867, 19.8345)
  line L1926 (-104.719, 57.9344) -> (-104.719, 52.1344)
  line L1927 (219.132, 33.0844) -> (219.929, 33.0844)
  line L1928 (161.467, 49.0338) -> (162.267, 49.0338)
  line L1929 (185.279, 10.9337) -> (186.08, 10.9337)
  line L1930 (185.279, 41.9836) -> (185.279, 38.8844)
  line L1931 (5.618, 19.8345) -> (5.618, 22.9336)
  line L1932 (4.817, 19.8345) -> (5.618, 19.8345)
  line L1933 (186.08, 33.0844) -> (186.08, 38.8844)
  line L1934 (157.217, 49.0338) -> (158.018, 49.0338)
  line L1935 (224.18, 29.9838) -> (223.379, 29.9838)
  line L1936 (157.217, -5.0157) -> (158.018, -5.0157)
  line L1937 (162.267, 48.0333) -> (162.267, 49.0338)
  line L1938 (224.18, 28.9833) -> (224.18, 29.9838)
  line L1939 (192.356, 3.4138) -> (194.081, 3.4138)
  line L1940 (-103.92, 49.0338) -> (-104.719, 49.0338)
  line L1941 (158.018, -8.1163) -> (157.217, -8.1163)
  line L1942 (157.217, 62.034) -> (157.217, 61.0336)
  line L1943 (185.279, 14.0343) -> (185.279, 10.9337)
  line L1944 (-99.6701, 52.1344) -> (-99.6701, 57.9344)
  line L1945 (185.279, 33.0844) -> (185.279, 29.9838)
  line L1946 (223.379, 38.8844) -> (224.18, 38.8844)
  line L1947 (195.605, 3.8837) -> (194.804, 3.8837)
  line L1948 (-100.4691, 49.0338) -> (-99.6701, 49.0338)
  line L1949 (5.618, 22.9336) -> (5.618, 19.8345)
  line L1950 (195.605, 3.8837) -> (195.605, 4.8841)
  line L1951 (186.08, 41.9836) -> (186.08, 42.984)
  line L1952 (192.356, 4.3343) -> (189.054, 4.3343)
  line L1953 (223.379, 33.0844) -> (223.379, 29.9838)
  line L1954 (186.08, 10.9337) -> (185.279, 10.9337)
  line L1955 (158.018, 3.8837) -> (158.018, 0.7845)
  line L1956 (5.618, 19.8345) -> (4.817, 19.8345)
  line L1957 (200.879, 22.9336) -> (200.082, 22.9336)
  line L1958 (161.467, 61.0336) -> (162.267, 61.0336)
  line L1959 (200.082, 22.9336) -> (200.082, 23.934)
  line L1960 (-99.6701, 49.0338) -> (-100.4691, 49.0338)
  line L1961 (-103.92, 57.9344) -> (-104.719, 57.9344)
  line L1962 (200.082, 38.8844) -> (200.082, 33.0844)
  line L1963 (205.13, 19.8345) -> (205.13, 14.0343)
  line L1964 (224.18, 42.984) -> (224.18, 41.9836)
  line L1965 (162.267, 57.9344) -> (161.467, 57.9344)
  line L1966 (219.132, 38.8844) -> (219.929, 38.8844)
  line L1967 (205.13, 19.8345) -> (204.329, 19.8345)
  line L1968 (161.467, 57.9344) -> (161.467, 61.0336)
  line L1969 (224.18, 33.0844) -> (223.379, 33.0844)
  line L1970 (5.618, 22.9336) -> (4.817, 22.9336)
  line L1971 (4.817, 23.934) -> (4.817, 22.9336)
  line L1972 (158.018, 52.1344) -> (158.018, 49.0338)
  line L1973 (186.08, 9.9333) -> (186.08, 10.9337)
  line L1974 (157.217, 3.8837) -> (158.018, 3.8837)
  line L1975 (157.217, 0.7845) -> (158.018, 0.7845)
  line L1976 (219.132, 28.9833) -> (219.132, 29.9838)
  line L1977 (223.379, 41.9836) -> (224.18, 41.9836)
  line L1978 (158.018, 57.9344) -> (158.018, 61.0336)
  line L1979 (200.879, 22.9336) -> (200.879, 19.8345)
  line L1980 (-104.719, 49.0338) -> (-104.719, 48.0333)
  line L1981 (204.329, 22.9336) -> (205.13, 22.9336)
  line L1982 (200.082, 22.9336) -> (200.879, 22.9336)
  line L1983 (9.867, 22.9336) -> (9.067, 22.9336)
  line L1984 (200.082, 23.934) -> (200.082, 22.9336)
  line L1985 (223.379, 29.9838) -> (224.18, 29.9838)
  line L1986 (158.018, -8.1163) -> (158.018, -5.0157)
  line L1987 (219.929, 38.8844) -> (219.929, 41.9836)
  line L1988 (-104.719, 61.0336) -> (-103.92, 61.0336)
  line L1989 (9.867, 23.934) -> (9.867, 22.9336)
  line L1990 (157.217, 4.8841) -> (157.217, 3.8837)
  line L1991 (158.018, 0.7845) -> (158.018, 3.8837)
  line L1992 (4.817, 22.9336) -> (5.618, 22.9336)
  line L1993 (205.13, 22.9336) -> (204.329, 22.9336)
  line L1994 (157.217, -8.1163) -> (158.018, -8.1163)
  line L1995 (162.267, 57.9344) -> (162.267, 52.1344)
  line L1996 (157.217, 0.7845) -> (157.217, -5.0157)
  line L1997 (158.018, 61.0336) -> (158.018, 57.9344)
  line L1998 (219.929, 29.9838) -> (219.929, 33.0844)
  line L1999 (224.18, 33.0844) -> (224.18, 38.8844)
  line L2000 (9.067, 22.9336) -> (9.867, 22.9336)
  line L2001 (162.267, 49.0338) -> (161.467, 49.0338)
  line L2002 (186.08, 22.9336) -> (185.279, 22.9336)
  line L2003 (9.867, 22.9336) -> (9.867, 23.934)
  line L2004 (162.267, 0.7845) -> (162.267, -5.0157)
  line L2005 (219.132, 29.9838) -> (219.929, 29.9838)
  line L2006 (157.217, 3.8837) -> (157.217, 4.8841)
  line L2007 (42.406, 71.1844) -> (42.406, 68.0838)
  line L2008 (223.379, 38.8844) -> (223.379, 41.9836)
  line L2009 (224.18, 38.8844) -> (224.18, 33.0844)
  line L2010 (205.13, 23.934) -> (205.13, 22.9336)
  line L2011 (38.955, 71.1844) -> (38.955, 68.0838)
  line L2012 (176.267, 61.0336) -> (176.267, 62.034)
  line L2013 (162.267, 62.034) -> (162.267, 61.0336)
  line L2014 (162.267, -8.1163) -> (162.267, -9.1167)
  line L2015 (200.082, 23.934) -> (186.08, 23.934)
  line L2016 (158.018, -5.0157) -> (158.018, -8.1163)
  line L2017 (43.205, 76.9844) -> (43.205, 71.1844)
  line L2018 (223.379, 29.9838) -> (223.379, 33.0844)
  line L2019 (185.279, 22.9336) -> (185.279, 19.8345)
  line L2020 (161.467, 0.7845) -> (161.467, 3.8837)
  line L2021 (42.406, 68.0838) -> (42.406, 71.1844)
  line L2022 (185.279, 19.8345) -> (186.08, 19.8345)
  line L2023 (223.379, 33.0844) -> (224.18, 33.0844)
  line L2024 (205.13, 42.984) -> (205.13, 41.9836)
  line L2025 (161.467, -8.1163) -> (162.267, -8.1163)
  line L2026 (200.082, 19.8345) -> (200.879, 19.8345)
  line L2027 (185.279, 22.9336) -> (186.08, 22.9336)
  line L2028 (186.08, 23.934) -> (186.08, 22.9336)
  line L2029 (224.18, 38.8844) -> (223.379, 38.8844)
  line L2030 (42.406, 80.0836) -> (42.406, 76.9844)
  line L2031 (161.467, 3.8837) -> (162.267, 3.8837)
  line L2032 (43.205, 81.084) -> (43.205, 80.0836)
  line L2033 (157.217, -5.0157) -> (157.217, 0.7845)
  line L2034 (224.18, 29.9838) -> (224.18, 28.9833)
  line L2035 (204.329, 33.0844) -> (204.329, 29.9838)
  line L2036 (162.267, 3.8837) -> (161.467, 3.8837)
  line L2037 (219.132, 29.9838) -> (219.132, 28.9833)
  line L2038 (42.406, 76.9844) -> (43.205, 76.9844)
  line L2039 (205.13, 38.8844) -> (205.13, 33.0844)
  line L2040 (195.605, 0.7845) -> (195.605, 0.1836)
  line L2041 (38.955, 76.9844) -> (38.955, 80.0836)
  line L2042 (-3.907, 41.9836) -> (-3.907, 38.8844)
  line L2043 (176.267, 62.034) -> (176.267, 61.0336)
  line L2044 (42.406, 71.1844) -> (43.205, 71.1844)
  line L2045 (205.13, 28.9833) -> (219.132, 28.9833)
  line L2046 (-4.708, 42.984) -> (-4.708, 41.9836)
  line L2047 (205.13, 29.9838) -> (205.13, 28.9833)
  line L2048 (204.329, 38.8844) -> (204.329, 41.9836)
  line L2049 (200.879, 38.8844) -> (200.879, 41.9836)
  line L2050 (189.054, -8.8866) -> (187.329, -8.8866)
  line L2051 (204.329, 41.9836) -> (204.329, 38.8844)
  line L2052 (-3.907, 29.9838) -> (-3.907, 33.0844)
  line L2053 (186.08, 23.934) -> (200.082, 23.934)
  line L2054 (157.217, -8.1163) -> (157.217, -9.1167)
  line L2055 (-3.907, 41.9836) -> (-4.708, 41.9836)
  line L2056 (162.267, 52.1344) -> (162.267, 57.9344)
  line L2057 (162.267, -5.0157) -> (161.467, -5.0157)
  line L2058 (176.267, 52.1344) -> (176.267, 57.9344)
  line L2059 (158.018, 3.8837) -> (157.217, 3.8837)
  line L2060 (-3.907, 38.8844) -> (-4.708, 38.8844)
  line L2061 (204.329, 19.8345) -> (205.13, 19.8345)
  line L2062 (157.217, -9.1167) -> (157.217, -8.1163)
  line L2063 (186.507, -2.6165) -> (187.329, -2.6165)
  line L2064 (200.082, 41.9836) -> (200.879, 41.9836)
  line L2065 (43.205, 68.0838) -> (43.205, 67.0833)
  line L2066 (219.132, 42.984) -> (205.13, 42.984)
  line L2067 (205.13, 29.9838) -> (204.329, 29.9838)
  line L2068 (205.13, 42.984) -> (219.132, 42.984)
  line L2069 (186.08, 19.8345) -> (186.08, 14.0343)
  line L2070 (194.804, 0.7845) -> (195.605, 0.7845)
  line L2071 (204.329, 19.8345) -> (204.329, 22.9336)
  line L2072 (219.132, 28.9833) -> (205.13, 28.9833)
  line L2073 (177.068, 52.1344) -> (177.068, 49.0338)
  line L2074 (185.279, 19.8345) -> (185.279, 22.9336)
  line L2075 (177.068, 57.9344) -> (176.267, 57.9344)
  line L2076 (-4.708, 41.9836) -> (-4.708, 42.984)
  line L2077 (176.267, 49.0338) -> (176.267, 48.0333)
  line L2078 (219.132, 10.9337) -> (219.132, 9.9333)
  line L2079 (205.13, 33.0844) -> (205.13, 38.8844)
  line L2080 (176.267, 57.9344) -> (177.068, 57.9344)
  line L2081 (186.507, 0.1836) -> (187.329, 0.1836)
  line L2082 (219.132, 9.9333) -> (219.132, 10.9337)
  line L2083 (-3.907, 29.9838) -> (-4.708, 29.9838)
  line L2084 (186.08, 19.8345) -> (185.279, 19.8345)
  line L2085 (176.267, 49.0338) -> (177.068, 49.0338)
  line L2086 (-4.708, 28.9833) -> (-4.708, 29.9838)
  line L2087 (205.13, 22.9336) -> (205.13, 23.934)
  line L2088 (-4.708, 38.8844) -> (-3.907, 38.8844)
  line L2089 (200.082, 38.8844) -> (200.879, 38.8844)
  line L2090 (192.356, -8.8866) -> (192.356, -9.8664)
  line L2091 (177.068, 61.0336) -> (177.068, 57.9344)
  line L2092 (-4.708, 33.0844) -> (-3.907, 33.0844)
  line L2093 (200.879, 41.9836) -> (200.082, 41.9836)
  line L2094 (200.082, 29.9838) -> (200.082, 28.9833)
  line L2095 (-94.395, 68.0838) -> (-94.395, 71.1844)
  line L2096 (200.082, 19.8345) -> (200.082, 14.0343)
  line L2097 (189.054, -9.8664) -> (189.054, -8.8866)
  line L2098 (-90.9441, 71.1844) -> (-90.1451, 71.1844)
  line L2099 (187.329, -8.8866) -> (187.329, -2.6165)
  line L2100 (186.08, 22.9336) -> (186.08, 23.934)
  line L2101 (200.879, 19.8345) -> (200.879, 22.9336)
  line L2102 (195.605, -8.1163) -> (194.804, -8.1163)
  line L2103 (-4.708, 33.0844) -> (-4.708, 38.8844)
  line L2104 (219.132, 14.0343) -> (219.132, 19.8345)
  line L2105 (177.068, 49.0338) -> (176.267, 49.0338)
  line L2106 (-90.9441, 76.9844) -> (-90.1451, 76.9844)
  line L2107 (-4.708, 41.9836) -> (-3.907, 41.9836)
  line L2108 (-3.907, 33.0844) -> (-4.708, 33.0844)
  line L2109 (192.356, -9.8664) -> (189.054, -9.8664)
  line L2110 (200.879, 33.0844) -> (200.082, 33.0844)
  line L2111 (200.879, 19.8345) -> (200.082, 19.8345)
  line L2112 (204.329, 29.9838) -> (205.13, 29.9838)
  line L2113 (176.267, 48.0333) -> (176.267, 49.0338)
  line L2114 (177.068, -5.0157) -> (177.068, -8.1163)
  line L2115 (-4.708, 38.8844) -> (-4.708, 33.0844)
  line L2116 (-90.1451, 67.0833) -> (-90.1451, 68.0838)
  line L2117 (200.082, 14.0343) -> (200.082, 19.8345)
  line L2118 (194.804, -5.0157) -> (195.605, -5.0157)
  line L2119 (194.081, -8.8866) -> (192.356, -8.8866)
  line L2120 (186.08, 14.0343) -> (186.08, 19.8345)
  line L2121 (177.068, 49.0338) -> (177.068, 52.1344)
  line L2122 (176.267, 52.1344) -> (177.068, 52.1344)
  line L2123 (219.132, 23.934) -> (219.132, 22.9336)
  line L2124 (-94.395, 71.1844) -> (-94.395, 68.0838)
  line L2125 (-90.9441, 76.9844) -> (-90.9441, 80.0836)
  line L2126 (205.13, 14.0343) -> (205.13, 19.8345)
  line L2127 (189.054, -8.8866) -> (189.054, -9.8664)
  line L2128 (-3.907, 38.8844) -> (-3.907, 41.9836)
  line L2129 (195.605, -4.4162) -> (195.605, -5.0157)
  line L2130 (-4.708, 29.9838) -> (-4.708, 28.9833)
  line L2131 (177.068, 3.8837) -> (177.068, 0.7845)
  line L2132 (-90.1451, 71.1844) -> (-90.1451, 76.9844)
  line L2133 (177.068, 61.0336) -> (176.267, 61.0336)
  line L2134 (204.329, 22.9336) -> (204.329, 19.8345)
  line L2135 (177.068, 3.8837) -> (176.267, 3.8837)
  line L2136 (176.267, 57.9344) -> (176.267, 52.1344)
  line L2137 (-90.1451, 68.0838) -> (-90.1451, 67.0833)
  line L2138 (-90.1451, 80.0836) -> (-90.9441, 80.0836)
  line L2139 (162.267, 49.0338) -> (162.267, 48.0333)
  line L2140 (176.267, 3.8837) -> (177.068, 3.8837)
  line L2141 (187.329, -2.6165) -> (186.507, -2.6165)
  line L2142 (-90.1451, 71.1844) -> (-90.9441, 71.1844)
  line L2143 (194.804, -5.0157) -> (194.804, -8.1163)
  line L2144 (162.267, -5.0157) -> (162.267, 0.7845)
  line L2145 (194.081, -4.4162) -> (195.605, -4.4162)
  line L2146 (195.605, 0.1836) -> (194.081, 0.1836)
  line L2147 (-90.1451, 76.9844) -> (-90.9441, 76.9844)
  line L2148 (-9.983, 22.9336) -> (-9.983, 19.8345)
  line L2149 (-3.907, 33.0844) -> (-3.907, 29.9838)
  line L2150 (176.267, -9.1167) -> (176.267, -8.1163)
  line L2151 (-90.1451, 76.9844) -> (-90.1451, 71.1844)
  line L2152 (176.267, -8.1163) -> (176.267, -9.1167)
  line L2153 (162.267, -9.1167) -> (162.267, -8.1163)
  line L2154 (-90.1451, 68.0838) -> (-90.9441, 68.0838)
  line L2155 (186.507, -2.6165) -> (186.507, 0.1836)
  line L2156 (-90.9441, 68.0838) -> (-90.9441, 71.1844)
  line L2157 (177.068, 52.1344) -> (176.267, 52.1344)
  line L2158 (209.607, -9.1167) -> (195.605, -9.1167)
  line L2159 (-4.708, 29.9838) -> (-3.907, 29.9838)
  line L2160 (194.804, -8.1163) -> (194.804, -5.0157)
  line L2161 (-90.1451, 80.0836) -> (-90.1451, 81.084)
  line L2162 (186.507, 0.1836) -> (186.507, -2.6165)
  line L2163 (177.068, 0.7845) -> (177.068, 3.8837)
  line L2164 (187.329, -2.6165) -> (187.329, -8.8866)
  line L2165 (192.356, -9.8664) -> (192.356, -8.8866)
  line L2166 (-90.9441, 68.0838) -> (-90.1451, 68.0838)
  line L2167 (219.929, 10.9337) -> (219.132, 10.9337)
  line L2168 (200.879, 29.9838) -> (200.082, 29.9838)
  line L2169 (195.605, 0.7845) -> (194.804, 0.7845)
  line L2170 (187.329, 0.1836) -> (186.507, 0.1836)
  line L2171 (219.929, 10.9337) -> (219.929, 14.0343)
  line L2172 (176.267, -5.0157) -> (176.267, 0.7845)
  line L2173 (-14.233, 19.8345) -> (-13.432, 19.8345)
  line L2174 (219.132, 10.9337) -> (219.929, 10.9337)
  line L2175 (-90.9441, 71.1844) -> (-90.9441, 68.0838)
  line L2176 (194.081, 0.1836) -> (195.605, 0.1836)
  line L2177 (194.081, -8.8866) -> (194.081, -4.4162)
  line L2178 (-90.9441, 80.0836) -> (-90.9441, 76.9844)
  line L2179 (224.18, 14.0343) -> (224.18, 19.8345)
  line L2180 (43.205, 68.0838) -> (42.406, 68.0838)
  line L2181 (194.081, -4.4162) -> (194.081, -8.8866)
  line L2182 (176.267, -5.0157) -> (177.068, -5.0157)
  line L2183 (177.068, -8.1163) -> (176.267, -8.1163)
  line L2184 (-94.395, 76.9844) -> (-94.395, 80.0836)
  line L2185 (219.132, 14.0343) -> (219.929, 14.0343)
  line L2186 (194.804, -8.1163) -> (195.605, -8.1163)
  line L2187 (219.929, 22.9336) -> (219.132, 22.9336)
  line L2188 (219.929, 19.8345) -> (219.132, 19.8345)
  line L2189 (195.605, -5.0157) -> (194.804, -5.0157)
  line L2190 (219.929, 22.9336) -> (219.929, 19.8345)
  line L2191 (-13.432, 22.9336) -> (-14.233, 22.9336)
  line L2192 (177.068, 0.7845) -> (176.267, 0.7845)
  line L2193 (223.379, 19.8345) -> (224.18, 19.8345)
  line L2194 (187.329, -8.8866) -> (189.054, -8.8866)
  line L2195 (162.267, 4.8841) -> (162.267, 3.8837)
  line L2196 (-14.233, 22.9336) -> (-14.233, 23.934)
  line L2197 (43.205, 80.0836) -> (42.406, 80.0836)
  line L2198 (223.379, 22.9336) -> (224.18, 22.9336)
  line L2199 (189.054, -9.8664) -> (192.356, -9.8664)
  line L2200 (38.955, 68.0838) -> (38.955, 71.1844)
  line L2201 (176.267, 3.8837) -> (176.267, 4.8841)
  line L2202 (-9.183, 22.9336) -> (-9.183, 23.934)
  line L2203 (177.068, 57.9344) -> (177.068, 61.0336)
  line L2204 (177.068, -8.1163) -> (177.068, -5.0157)
  line L2205 (204.329, 33.0844) -> (205.13, 33.0844)
  line L2206 (-90.9441, 80.0836) -> (-90.1451, 80.0836)
  line L2207 (-90.1451, 81.084) -> (-90.1451, 80.0836)
  line L2208 (224.18, 23.934) -> (224.18, 22.9336)
  line L2209 (224.18, 10.9337) -> (223.379, 10.9337)
  line L2210 (192.356, -8.8866) -> (194.081, -8.8866)
  line L2211 (195.605, -8.1163) -> (195.605, -9.1167)
  line L2212 (-14.233, 22.9336) -> (-13.432, 22.9336)
  line L2213 (176.267, 62.034) -> (162.267, 62.034)
  line L2214 (-9.183, 22.9336) -> (-9.983, 22.9336)
  line L2215 (176.267, -8.1163) -> (177.068, -8.1163)
  line L2216 (224.18, 14.0343) -> (223.379, 14.0343)
  line L2217 (-14.233, 23.934) -> (-14.233, 22.9336)
  line L2218 (205.13, 41.9836) -> (204.329, 41.9836)
  line L2219 (-94.395, 80.0836) -> (-94.395, 76.9844)
  line L2220 (-13.432, 19.8345) -> (-13.432, 22.9336)
  line L2221 (176.267, 61.0336) -> (177.068, 61.0336)
  line L2222 (176.267, 0.7845) -> (177.068, 0.7845)
  line L2223 (176.267, 0.7845) -> (176.267, -5.0157)
  line L2224 (42.406, 68.0838) -> (43.205, 68.0838)
  line L2225 (195.605, -4.4162) -> (194.081, -4.4162)
  line L2226 (224.18, 19.8345) -> (224.18, 14.0343)
  line L2227 (200.879, 33.0844) -> (200.879, 29.9838)
  line L2228 (223.379, 22.9336) -> (223.379, 19.8345)
  line L2229 (204.329, 29.9838) -> (204.329, 33.0844)
  line L2230 (-9.183, 19.8345) -> (-9.983, 19.8345)
  line L2231 (200.879, 41.9836) -> (200.879, 38.8844)
  line L2232 (176.267, 4.8841) -> (176.267, 3.8837)
  line L2233 (224.18, 10.9337) -> (224.18, 9.9333)
  line L2234 (224.18, 19.8345) -> (223.379, 19.8345)
  line L2235 (-13.432, 19.8345) -> (-14.233, 19.8345)
  line L2236 (-13.432, 22.9336) -> (-13.432, 19.8345)
  line L2237 (162.267, 3.8837) -> (162.267, 4.8841)
  line L2238 (177.068, -5.0157) -> (176.267, -5.0157)
  line L2239 (162.267, 48.0333) -> (176.267, 48.0333)
  line L2240 (162.267, 62.034) -> (176.267, 62.034)
  line L2241 (176.267, -9.1167) -> (162.267, -9.1167)
  line L2242 (-9.983, 19.8345) -> (-9.983, 22.9336)
  line L2243 (205.13, 33.0844) -> (204.329, 33.0844)